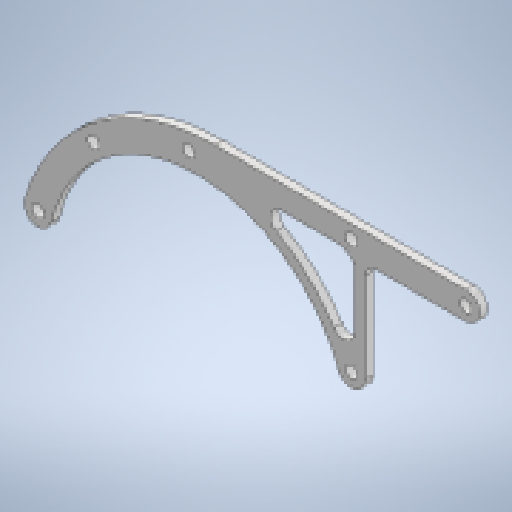
# Autodesk Inventor part: tesaki
Saved by Autodesk Inventor 2025.1 (Build 291241000, 241)
## iProperties
Created: 2024-09-04
Part Number: tesaki
Material: アルミニウム 2014-T4
Document SubType Name: Modeling
Designer: right
Mass: 2.35989 g
Surface Area: 16.1484 cm^2
Volume: 0.842818 cm^3
Density: 2.8 g/cm^3
Appearance: サテン
Author: right
Autodesk Inventor part; units mm, degrees
ref_plane "YZ Plane" through (0, 0, 0) normal (1, 0, 0) x (0, 1, 0)
ref_plane "XZ Plane" through (0, 0, 0) normal (0, 1, 0) x (-1, 0, 0)
ref_plane "XY Plane" through (0, 0, 0) normal (0, 0, 1) x (1, 0, 0)
sketch "スケッチ2" plane through (0, 0, 0) normal (0, 0, 1) x (1, 0, 0)
  circle A0 centre (24.8946, 24.5696) radius 0.85 projected
  circle A1 centre (3.8946, 24.5696) radius 0.85 projected
  circle A2 centre (3.8946, 3.5696) radius 0.85 projected
  circle A3 centre (24.8946, 24.5696) radius 2.5
  circle A4 centre (24.8946, 24.5696) radius 1.1
  circle A5 centre (3.8946, 24.5696) radius 1.1
  circle A6 centre (3.8946, 24.5696) radius 2.5
  circle A7 centre (3.8946, 3.5696) radius 2.5
  circle A8 centre (3.8946, 3.5696) radius 1.1
  line L0 (24.8946, 27.0696) -> (3.8946, 27.0696)
  line L1 (24.8946, 22.0696) -> (3.8946, 22.0696)
  line L2 (6.3946, 24.5696) -> (6.3946, 3.5696)
  line L3 (3.8946, 27.0696) -> (-21.1054, 27.0696)
  arc A9 (-21.1054, 27.0696) -> (-56.0009, 1.0696) centre (-21.1054, -9.3477) ccw
  line L4 (3.8946, 1.0696) -> (-56.0009, 1.0696) construction
  circle A10 centre (-53.6054, 0.3545) radius 2.5
  arc A11 (1.5492, 2.7041) -> (-51.1781, -0.2441) centre (-24.3623, -6.8571) ccw
  circle A12 centre (-25.9042, 23.7232) radius 3 construction
  circle A13 centre (-53.6054, 0.3545) radius 1.1
  circle A14 centre (-25.9042, 23.7232) radius 1.1
  circle A15 centre (-43.3948, 16.3537) radius 2.3971 construction
  line L5 (-43.3948, 16.3537) -> (-25.9042, 23.7232) construction
  line L6 (-43.3948, 16.3537) -> (-53.6054, 0.3545) construction
  circle A16 centre (-43.3948, 16.3537) radius 1.1
  point P0 (0, 0)
  point P1 (3.8946, 1.0696)
  point P2 (1.4587, 3.0071)
  point P3 (-51.2099, 1.0696)
  point P4 (-55.9852, 1.6541)
  point P5 (6.3946, 22.0696)
  point P6 (-25.9042, 20.719)
  dimension "d10" = 5
  dimension "d11" = 2.2
  dimension "d12" = 2.2
  dimension "d13" = 5
  dimension "d14" = 5
  dimension "d15" = 2.2
  dimension "d16" = 25
  dimension "d17" = 5
  dimension "d21" = 60
  dimension "d23" = 6
  dimension "d24" = 2.2
  dimension "d25" = 2.2
  dimension "d26" = 2.2
  constraints: 17 point on circle, 14 centre point, 14 tangent, 12 end point, 9 coincident, 1 equal length, 1 point on line, 1 vertical alignment, 5 other
  measures "d10" diameter of A3
  measures "d11" diameter of A4
  measures "d12" diameter of A5
  measures "d13" diameter of A6
  measures "d14" diameter of A7
  measures "d15" diameter of A8
  measures "d16" distance of L0.end L3.end
  measures "d17" diameter of A10
  measures "d21" distance from line of L2 A10.centre
  measures "d23" diameter of A12
  measures "d24" diameter of A13
  measures "d25" diameter of A14
  measures "d26" diameter of A16
extrude "押し出し1" add sketch "スケッチ2" along normal blind 1.5 contours A3 | A3 L1 L2 A6 L0 | A6 | A6 L1 L2 A7 A11 A10 A9 L3 | L1 A6 L2 | A7 | A10
fillet "フィレット1" radius 2 1 edges at (6.3946, 22.0696, 0.75)
sketch "スケッチ3" plane through (0, 0, 1.5) normal (0, 0, 1) x (1, 0, 0)
  line L0 (-24.3623, 22.7621) -> (4.3946, 22.7621)
  line L1 (4.3946, 22.7621) -> (4.3946, 6.0191)
  line L2 (6.3946, 3.5696) -> (6.3946, 20.0696) projected
  line L3 (24.8946, 27.0696) -> (-21.1054, 27.0696) projected
  circle A0 centre (3.8946, 24.5696) radius 1.1 projected
  circle A1 centre (3.8946, 24.5696) radius 2.5
  arc A2 (1.5492, 2.7041) -> (-51.1781, -0.2441) centre (-24.3623, -6.8571) ccw projected
  arc A3 (1.5492, 2.7041) -> (6.3946, 3.5696) centre (3.8946, 3.5696) ccw projected
  circle A4 centre (3.8946, 3.5696) radius 2.5
  arc A5 (3.4255, 3.3965) -> (-53.12, 0.2347) centre (-24.3623, -6.8571) ccw
  arc A6 (3.4255, 3.3965) -> (4.3946, 3.5696) centre (3.8946, 3.5696) ccw
  line L4 (4.3946, 3.5696) -> (4.3946, 20.0696)
  point P0 (0, 0)
  point P1 (2.4919, 5.639)
  point P2 (4.3946, 22.1201)
  point P3 (2.1675, 22.7621)
  dimension "d27" = 2
  dimension "d30" = 2
  constraints: 7 point on circle, 6 end point, 4 centre point, 2 coincident, 2 tangent, 1 horizontal, 1 perpendicular, 2 other
  measures "d27" distance between parallel lines of L2 L1
  measures "d30" radial gap between concentric circles of A2 A5
extrude "押し出し2" cut sketch "スケッチ3" against normal through all contours L0 A1 L1 A4 A5
fillet "フィレット2" radius 2 5 edges at (-24.3623, 22.7621, 0.75) (2.4919, 5.639, 0.75) (4.3946, 6.0191, 0.75) (4.3946, 22.1201, 0.75) (2.1675, 22.7621, 0.75)
sketch "スケッチ4" plane through (0, 0, 1.5) normal (0, 0, 1) x (1, 0, 0)
  circle A0 centre (-15.7592, 24.9158) radius 1.1
  circle A1 centre (-0.7592, 24.9158) radius 1.1
  circle A2 centre (-0.7592, 24.9158) radius 2.1538
  line L0 (24.8946, 27.0696) -> (-21.1054, 27.0696) projected
  line L1 (-8.969, 22.7621) -> (1.4961, 22.7621) projected
  line L2 (1.3946, 24.5696) -> (1.3946, 3.5696) projected
  point P0 (0, 0)
  dimension "d34" = 2.2
  dimension "d35" = 2.2
  dimension "d36" = 15
  constraints: 3 centre point, 3 tangent, 1 coincident, 1 horizontal alignment
  measures "d34" diameter of A0
  measures "d35" diameter of A1
  measures "d36" distance of A1.centre A0.centre
extrude "押し出し3" cut sketch "スケッチ4" against normal through all contours A0 | A1
